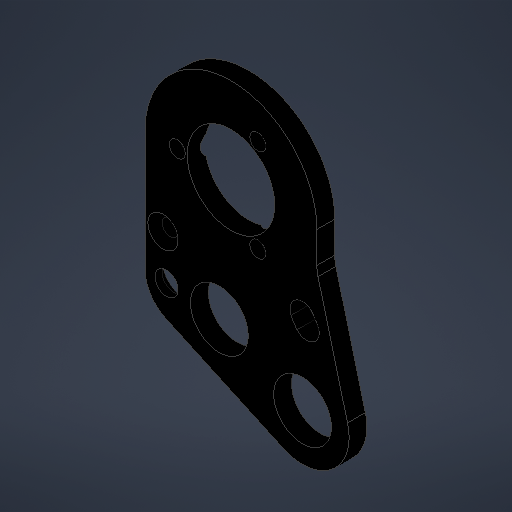
# Autodesk Inventor part: Dribbler Bracket
Saved by Autodesk Inventor 2026.1 (Build 301233020, 233B)
## iProperties
Created: 2025-12-14
Part Number: Dribbler Bracket
Material: Generic
Document SubType Name: Modeling
Designer: Bahaa
Density: 1 g/cm^3
Appearance: Default
Author: Bahaa
Autodesk Inventor part; units mm, degrees
ref_plane "YZ Plane" through (0, 0, 0) normal (1, 0, 0) x (0, 1, 0)
ref_plane "XZ Plane" through (0, 0, 0) normal (0, 1, 0) x (-1, 0, 0)
ref_plane "XY Plane" through (0, 0, 0) normal (0, 0, 1) x (1, 0, 0)
sketch "Sketch1" plane through (0, 0, 0) normal (0, 1, 0) x (-1, 0, 0)
  circle A0 centre (0, 0) radius 1.75 construction
  circle A1 centre (10, 11.472032) radius 12
  line L0 (0, 0) -> (10, 11.472032) construction
  line L1 (0, 0) -> (4, 0) construction
  circle A2 centre (0, 0) radius 4 construction
  circle A3 centre (0, -11.440846) radius 6.5
  line L2 (10, 11.472032) -> (0, -11.440846) construction
  line L3 (0, 0) -> (0, -11.440846) construction
  line L4 (0, 0) -> (0, -4) construction
  line L5 (22, 11.472032) -> (22, -8.527968)
  line L6 (22, -8.527968) -> (2.703128, -17.352115)
  line L7 (-2, 11.472032) -> (-2, 6.472032)
  line L8 (-2, 6.472032) -> (-6.285281, -9.783969)
  circle A4 centre (10, 11.472032) radius 9.55
  line L9 (10, 11.472032) -> (17.5, 11.472032) construction
  circle A5 centre (17.5, 11.472032) radius 1.1
  circle A6 centre (6.25, 17.967223) radius 1.1
  circle A7 centre (6.25, 4.976842) radius 1.1
  circle A8 centre (10, 11.472032) radius 6.1
  circle A9 centre (0, -11.440846) radius 4.025
  circle A10 centre (10, 11.472032) radius 10
  circle A11 centre (0, -11.440846) radius 5
  circle A12 centre (11.624641, -6.20346) radius 7.75
  circle A13 centre (11.624641, -6.20346) radius 4.025
  circle A14 centre (19, -5.527968) radius 1.6
  circle A15 centre (19.5, 0.472032) radius 1.35
  circle A16 centre (0, -11.440846) radius 5.5
  circle A17 centre (10, 11.472032) radius 10.5
  dimension "d5" = 8
  dimension "d0" = 3.5
  dimension "d1" = 24
  dimension "d2" = 4
  dimension "d4" = 10
  dimension "d6" = 13
  dimension "d7" = 25
  dimension "d8" = 17.5
  dimension "d12" = 0
  dimension "d13" = 20
  dimension "d14" = 5
  dimension "d17" = 19.1
  dimension "d19" = 7.5
  dimension "d20" = 2.2
  dimension "d23" = 360
  dimension "d25" = 12.2
  dimension "d26" = 8.05
  dimension "d38" = 20
  dimension "d39" = 10
  dimension "d40" = 15.5
  dimension "d41" = 8.05
  dimension "d42" = 3.2
  dimension "d43" = 3
  dimension "d44" = 3
  dimension "d53" = 2.5
  dimension "d54" = 9
  dimension "d56" = 2.7
  dimension "d67" = 11
  dimension "d69" = 21
  constraints: 20 end point, 17 centre point, 12 coincident, 6 tangent, 4 point on circle, 3 vertical, 2 horizontal, 1 vertical alignment, 9 other
  measures "d0" diameter of A0
  measures "d1" diameter of A1
  measures "d2" distance of L0.start L1.end
  measures "d4" horizontal distance of point (0, 0) L0.end
  measures "d6" diameter of A3
  measures "d7" distance of L0.end L2.end
  measures "d8" angle of L0 L2
  measures "d12" distance between parallel lines of L4 L3
  measures "d13" distance of L5.start L5.end
  measures "d14" distance of L7.start L7.end
  measures "d17" diameter of A4
  measures "d19" distance of L9.start L9.end
  measures "d20" diameter of A5
  measures "d25" diameter of A8
  measures "d26" diameter of A9
  measures "d38" diameter of A10
  measures "d39" diameter of A11
  measures "d40" diameter of A12
  measures "d41" diameter of A13
  measures "d42" diameter of A14
  measures "d43" distance from line of L5 A14.centre
  measures "d44" horizontal distance of L5.end A14.centre
  measures "d53" distance from line of L5 point (19.5, 0.472)
  measures "d54" vertical distance of L5.end point (19.5, 0.472)
  measures "d56" diameter of A15
  measures "d67" diameter of A16
  measures "d69" diameter of A17
sketch "Sketch1 outline for Extrusion1" plane through (0, 0, 0) normal (0, 1, 0) x (-1, 0, 0)
  circle A0 centre (10, 11.472032) radius 6.1
  line L0 (-2, 11.472032) -> (-2, 6.472032)
  line L1 (-2, 6.472032) -> (-6.285281, -9.783969)
  arc A1 (-6.285281, -9.783969) -> (2.703128, -17.352115) centre (0, -11.440846) ccw
  line L2 (2.703128, -17.352115) -> (22, -8.527968)
  line L3 (22, -8.527968) -> (22, 11.472032)
  arc A2 (22, 11.472032) -> (-2, 11.472032) centre (10, 11.472032) ccw
extrude "Extrusion1" add sketch "Sketch1 outline for Extrusion1" against normal blind 2.5
sketch "Sketch1 outline for Extrusion2" plane through (0, 0, 0) normal (0, 1, 0) x (-1, 0, 0)
  circle A0 centre (0, -11.440846) radius 4.025
  circle A1 centre (11.624641, -6.20346) radius 4.025
extrude "Extrusion2" cut sketch "Sketch1 outline for Extrusion2" against normal blind 2.5
hole "Hole1" at (-17.5, 0, 11.472032) at (-6.25, 0, 17.967223) at (-6.25, 0, 4.976842) direction (0, -1, 0) diameter 2.2 end through all countersink diameter 4.2 countersink angle 90
hole "Hole2" at (-19, 0, -5.527968) direction (0, -1, 0) diameter 3.2 end through all countersink diameter 6.2 countersink angle 90
fillet "Fillet1" radius 5 2 edges at (-22, -1.25, -8.528) (2, -1.25, 6.472)
sketch "Sketch3" plane through (0, -2.5, 0) normal (0, -1, 0) x (1, 0, 0)
  point P0 (0, 0)
  point P1 (-19.5, 0.472032)
hole "Hole3" at (-19.5, -2.5, 0.472032) direction (0, 1, 0) diameter 2.2 end through all countersink diameter 4.2 countersink angle 90
sketch "Sketch4" plane through (0, 0, 0) normal (0, 1, 0) x (1, 0, 0)
  circle A0 centre (0, 0) radius 1.75 construction
  circle A1 centre (0, 0) radius 4 construction
  line L0 (2, -1.472032) -> (3.318061, -1.472032) construction
  line L1 (6.285281, 9.783969) -> (2.165168, -5.845474)
  arc A2 (0.568061, 0.897337) -> (0, 0) centre (3.318061, -1.472032) ccw construction
  arc A3 (-0.757721, 2.039616) -> (-1.599646, 0.709671) centre (3.318061, -1.472032) ccw
  arc A4 (1.893843, -0.244942) -> (1.599646, -0.709671) centre (3.318061, -1.472032) ccw
  arc A5 (1.893843, -0.244942) -> (-0.757721, 2.039616) centre (0.568061, 0.897337) ccw
  arc A6 (-1.599646, 0.709671) -> (1.599646, -0.709671) centre (0, 0) ccw
  line L2 (2, -1.472032) -> (2, -6.472032) construction
  dimension "d74" = 2.75
  dimension "d80" = 5
  constraints: 10 point on circle, 5 centre point, 4 end point, 4 tangent, 2 coincident, 1 concentric, 1 perpendicular, 1 point on line, 1 vertical
  measures "d74" horizontal distance of L0.end A2.start
  measures "d80" distance of L2.start L2.end
extrude "Extrusion3" cut sketch "Sketch4" against normal blind 2.5
body "Solid1"
